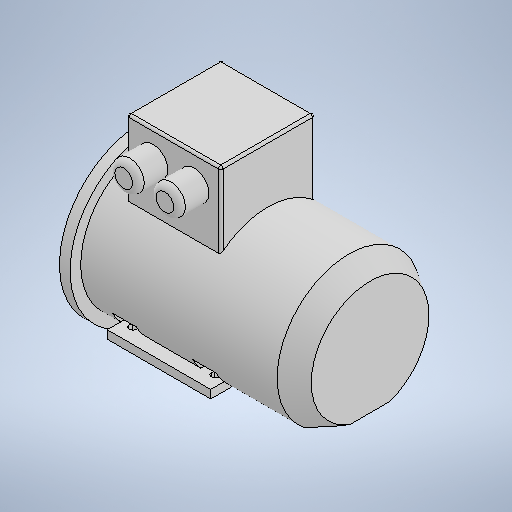
# Autodesk Inventor part: СДР 060 Мотор-редуктор 2.0
Saved by Autodesk Inventor 2025.1 (Build 291241020, 241B)
## iProperties
Created: 2024-04-02
Part Number: СДР 060 Мотор-редуктор 2.0
Material: Типовые
Document SubType Name: Modeling
Designer: pokla
Density: 1 g/cm^3
Appearance: По умолчанию
Author: pokla
Autodesk Inventor part; units mm, degrees
ref_plane "YZ Plane" through (0, 0, 0) normal (1, 0, 0) x (0, 1, 0)
ref_plane "XZ Plane" through (0, 0, 0) normal (0, 1, 0) x (-1, 0, 0)
ref_plane "XY Plane" through (0, 0, 0) normal (0, 0, 1) x (1, 0, 0)
sketch "Эскиз1" plane through (0, 0, 0) normal (0, 1, 0) x (-1, 0, 0)
  line L0 (0, 0) -> (0, -70)
  line L1 (0, -70) -> (-9, -70)
  line L2 (-9, -70) -> (-9, -61)
  line L3 (-9, -61) -> (-176, -61)
  line L4 (-176, -61) -> (-194, -50)
  line L5 (-194, -50) -> (-194, 0)
  line L6 (-194, 0) -> (0, 0)
  point P0 (-4.5, -70)
  dimension "d0" = 194
  dimension "d1" = 9
  dimension "d14" = 140
  dimension "d103" = 122
  dimension "d104" = 100
  dimension "d105" = 18
  constraints: 14 end point, 4 perpendicular, 1 midpoint, 1 parallel, 1 vertical
  measures "d0" distance of L5.end L0.start
  measures "d1" distance of L0.end L1.end
  measures "d14" diameter of point (-4.5, -70) L6
  measures "d103" diameter of L3 L6
  measures "d104" diameter of L4.end L6
  measures "d105" distance from line of L5 L3.end
revolve "Вращение1" add sketch "Эскиз1" angle 360 about axis through (194, 0, 0) along (-1, 0, 0)
sketch "Эскиз5" plane through (0, 0, 0) normal (0, 1, 0) x (-1, 0, 0)
  line L0 (-176, -61) -> (-176, 61) projected
  line L1 (-9, -61) -> (-9, 61) projected
  line L2 (-27, -40) -> (-107, -40)
  line L3 (-107, -40) -> (-107, 40)
  line L4 (-107, 40) -> (-27, 40)
  line L5 (-27, 40) -> (-27, -40)
  point P0 (0, 0)
  point P1 (-27, 0)
  point P2 (-9, 0)
  dimension "d38" = 80
  dimension "d40" = 18
  constraints: 8 end point, 2 midpoint, 2 parallel, 2 perpendicular, 1 horizontal, 1 horizontal alignment
  measures "d38" distance of L3.end L4.end
  measures "d40" distance between parallel lines of L1 L5
extrude "Выдавливание4" add sketch "Эскиз5" along normal blind 110
sketch "Sketch15" plane through (27, 46.0543, 40) normal (0, 0, 1) x (1, 0, 0)
  circle A0 centre (22.5, 39.9457) radius 12.5
  circle A1 centre (57.5, 39.9457) radius 12.5
  line L0 (80, 63.9457) -> (0, 63.9457) construction
  line L1 (40, 63.9457) -> (40, 0) construction
  line L2 (0, 0) -> (80, 0) construction
  point P0 (-27, -46.0543)
  dimension "d106" = 25
  dimension "d107" = 35
  dimension "d108" = 24
  constraints: 2 centre point, 2 end point, 2 midpoint, 1 equal radius, 1 horizontal alignment, 1 symmetric about line
  measures "d106" diameter of A0
  measures "d107" distance of A1.centre A0.centre
  measures "d108" distance from line of A0.centre L0
extrude "Extrusion14" add sketch "Sketch15" along normal blind 25
fillet "Fillet1" radius 5 2 edges at (37, 86, 65) (72, 86, 65)
fillet "Fillet2" radius 2 8 edges at (27, 78.0272, 40) (67, 110, 40) (107, 78.0272, 40) (107, 110, 0) (67, 110, -40) (27, 110, 0) (107, 78.0272, -40) (27, 78.0272, -40)
sketch "Sketch16" plane through (9, 0, 0) normal (1, 0, 0) x (0, 0, -1)
  circle A0 centre (0, 0) radius 61 projected
  line L0 (-38.8844, -47) -> (38.8844, -47)
  line L1 (0, -61) -> (0, -47) construction
  dimension "d113" = 14
  constraints: 4 end point, 3 point on circle, 1 horizontal, 1 midpoint, 1 vertical
  measures "d113" distance of L1.start L1.end
extrude "Extrusion15" cut sketch "Sketch16" along normal up to surface (185 mm away) contours L0 A0 picked at (-10.0748, -48.9953)
sketch "Sketch17" plane through (9, -47, -38.8844) normal (0, -1, 0) x (1, 0, 0)
  line L0 (0, 77.7689) -> (167, 77.7689) construction
  line L1 (0, 0) -> (0, 77.7689) construction
  line L2 (167, 0) -> (0, 0) construction
  line L3 (185, 55.9432) -> (185, 21.8257) construction
  line L4 (19, -18.6156) -> (107, -18.6156)
  line L5 (107, -18.6156) -> (107, 96.3844)
  line L6 (107, 96.3844) -> (19, 96.3844)
  line L7 (19, 96.3844) -> (19, -18.6156)
  line L8 (19, -18.6156) -> (107, 96.3844) construction
  line L9 (107, -18.6156) -> (19, 96.3844) construction
  line L10 (28, 80.8844) -> (28, 83.8844) construction
  line L11 (25, 80.8844) -> (25, 83.8844)
  line L12 (31, 83.8844) -> (31, 80.8844)
  arc A0 (25, 80.8844) -> (31, 80.8844) centre (28, 80.8844) ccw
  arc A1 (31, 83.8844) -> (25, 83.8844) centre (28, 83.8844) ccw
  line L13 (98, 80.8844) -> (98, 83.8844) construction
  line L14 (101, 80.8844) -> (101, 83.8844)
  line L15 (95, 83.8844) -> (95, 80.8844)
  arc A2 (95, 80.8844) -> (101, 80.8844) centre (98, 80.8844) ccw
  arc A3 (101, 83.8844) -> (95, 83.8844) centre (98, 83.8844) ccw
  line L16 (98, -6.1156) -> (98, -3.1156) construction
  line L17 (101, -6.1156) -> (101, -3.1156)
  line L18 (95, -3.1156) -> (95, -6.1156)
  arc A4 (95, -6.1156) -> (101, -6.1156) centre (98, -6.1156) ccw
  arc A5 (101, -3.1156) -> (95, -3.1156) centre (98, -3.1156) ccw
  line L19 (28, -6.1156) -> (28, -3.1156) construction
  line L20 (31, -6.1156) -> (31, -3.1156)
  line L21 (25, -3.1156) -> (25, -6.1156)
  arc A6 (25, -6.1156) -> (31, -6.1156) centre (28, -6.1156) ccw
  arc A7 (31, -3.1156) -> (25, -3.1156) centre (28, -3.1156) ccw
  line L22 (-9, 108.8844) -> (-9, -31.1156) projected
  line L23 (63, 38.8844) -> (-9, 38.8844) construction
  point P0 (28, 82.3844)
  point P1 (98, 82.3844)
  point P2 (98, -4.6156)
  point P3 (28, -4.6156)
  dimension "d116" = 115
  dimension "d117" = 88
  dimension "d118" = 37
  dimension "d119" = 70
  dimension "d120" = 28
  dimension "d121" = 3
  dimension "d122" = 3
  dimension "d123" = 14
  constraints: 46 end point, 16 point on circle, 16 tangent, 8 centre point, 7 parallel, 6 midpoint, 3 equal length, 3 perpendicular, 2 horizontal alignment, 2 point on line, 1 collinear, 1 equal radius, 1 horizontal, 4 other
  measures "d116" distance of L6.end L4.start
  measures "d117" distance of L5.end L6.end
  measures "d118" distance between parallel lines of L10 L22
  measures "d119" distance between parallel lines of L10 L13
  measures "d120" distance between parallel lines of L7 L22
  measures "d121" radius of A0
  measures "d122" distance of L10.start L10.end
  measures "d123" distance from line of L6 point (28, 82.384)
extrude "Extrusion16" add sketch "Sketch17" against normal blind 7
sketch "Sketch18" plane through (28, -47, 38.8844) normal (-1, 0, 0) x (0, 0, 1)
  line L0 (18.6156, 0) -> (18.6156, 7) projected
  line L1 (-96.3844, 0) -> (-96.3844, 7) projected
  line L2 (-96.3844, 7) -> (18.6156, 7)
  line L3 (-84.9388, 7) -> (-96.3844, 7) projected
  line L4 (18.6156, 7) -> (-1.3844, 7)
  line L5 (-1.3844, 7) -> (-1.3844, 17)
  line L6 (-1.3844, 17) -> (18.6156, 17)
  line L7 (18.6156, 17) -> (18.6156, 7)
  line L8 (-96.3844, 7) -> (-76.3844, 7)
  line L9 (-76.3844, 7) -> (-76.3844, 17)
  line L10 (-76.3844, 17) -> (-96.3844, 17)
  line L11 (-96.3844, 17) -> (-96.3844, 7)
  point P0 (-38.8844, 47)
  point P1 (-76.3844, 7)
  point P2 (-1.3844, 7)
  dimension "d126" = 20
  dimension "d127" = 10
  constraints: 18 end point, 4 parallel, 2 equal length, 2 horizontal, 2 perpendicular, 1 collinear
  measures "d126" distance of L5.end L6.end
  measures "d127" distance of L4.end L5.end
extrude "Extrusion17" cut sketch "Sketch18" against normal blind 20
pattern_linear "Rectangular Pattern2" count 2 spacing 68 along (1, 0, 0) of "Extrusion17"
sketch "Sketch19" plane through (9, -47, -38.8844) normal (0, -1, 0) x (1, 0, 0)
  arc A0 (95, -6.1156) -> (101, -6.1156) centre (98, -6.1156) ccw projected
  line L0 (95, -6.1156) -> (95, -3.1156) projected
  arc A1 (101, -3.1156) -> (95, -3.1156) centre (98, -3.1156) ccw projected
  line L1 (101, -3.1156) -> (101, -6.1156) projected
  arc A2 (25, -6.1156) -> (31, -6.1156) centre (28, -6.1156) ccw projected
  line L2 (25, -6.1156) -> (25, -3.1156) projected
  arc A3 (31, -3.1156) -> (25, -3.1156) centre (28, -3.1156) ccw projected
  line L3 (31, -3.1156) -> (31, -6.1156) projected
  arc A4 (95, 80.8844) -> (101, 80.8844) centre (98, 80.8844) ccw projected
  line L4 (95, 80.8844) -> (95, 83.8844) projected
  arc A5 (101, 83.8844) -> (95, 83.8844) centre (98, 83.8844) ccw projected
  line L5 (101, 83.8844) -> (101, 80.8844) projected
  line L6 (31, 83.8844) -> (31, 80.8844) projected
  arc A6 (25, 80.8844) -> (31, 80.8844) centre (28, 80.8844) ccw projected
  line L7 (25, 80.8844) -> (25, 83.8844) projected
  arc A7 (31, 83.8844) -> (25, 83.8844) centre (28, 83.8844) ccw projected
  line L8 (0, 77.7689) -> (19, 77.7689) projected
  line L9 (0, 0) -> (0, 77.7689) projected
  line L10 (19, 0) -> (0, 0) projected
  line L11 (19, 0) -> (19, -18.6156) projected
  line L12 (19, -18.6156) -> (107, -18.6156) projected
  line L13 (107, -18.6156) -> (107, 0) projected
  line L14 (167, 0) -> (107, 0) projected
  line L15 (185, 55.9432) -> (185, 21.8257) projected
  line L16 (107, 77.7689) -> (167, 77.7689) projected
  line L17 (107, 77.7689) -> (107, 96.3844) projected
  line L18 (107, 96.3844) -> (19, 96.3844) projected
  line L19 (19, 96.3844) -> (19, 77.7689) projected
  point P0 (-9, 38.8844)
  constraints: 2 other
extrude "Extrusion18" cut sketch "Sketch19" against normal blind 10
equation "\"Reductor_angle\" = 180deg"
